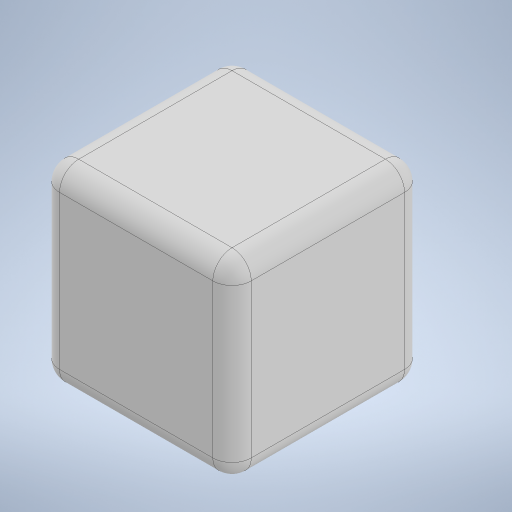
# Autodesk Inventor part: Holder
Saved by Autodesk Inventor 2023 (Build 270158000, 158)
## iProperties
Created: 2022-12-13
Part Number: Holder
Material: Generic
Document SubType Name: Modeling
Designer: romanp
Density: 1 g/cm^3
Appearance: Default
Author: romanp
Autodesk Inventor part; units mm, degrees
ref_plane "YZ Plane" through (0, 0, 0) normal (1, 0, 0) x (0, 1, 0)
ref_plane "XZ Plane" through (0, 0, 0) normal (0, 1, 0) x (-1, 0, 0)
ref_plane "XY Plane" through (0, 0, 0) normal (0, 0, 1) x (1, 0, 0)
sketch "Sketch5" plane through (0, 0, 0) normal (0, 0, 1) x (1, 0, 0)
  circle A0 centre (0, 0) radius 3.75
  dimension "d11" = 7.5
  constraints: 1 centre point, 1 coincident
  measures "d11" diameter of A0
extrude "Extrusion4" add sketch "Sketch5" along normal blind 5
sketch "Sketch6" plane through (0, 0, 5) normal (0, 0, 1) x (1, 0, 0)
  line L0 (0, 0) -> (-10, 0)
  line L1 (-10, 0) -> (-10, 10)
  line L2 (-10, 10) -> (10, 10)
  line L3 (10, 10) -> (10, -10)
  line L4 (10, -10) -> (-10, -10)
  line L5 (-10, -10) -> (-10, 0)
  dimension "d19" = 10
  dimension "d20" = 10
  dimension "d21" = 20
  dimension "d22" = 20
  dimension "d23" = 20
  constraints: 12 end point, 3 perpendicular, 1 collinear, 1 horizontal, 1 point on line
  measures "d19" distance of L0.start L0.end
  measures "d20" distance of L0.end L1.end
  measures "d21" distance of L1.end L2.end
  measures "d22" distance of L2.end L3.end
  measures "d23" distance of L3.end L4.end
extrude "Extrusion5" add sketch "Sketch6" along normal blind 20
fillet "Fillet1" radius 2 12 edges at (-10, 0, 5) (0, -10, 5) (-10, -10, 15) (0, 10, 5) (10, 10, 15) (10, 0, 5) (-10, 10, 15) (-10, 0, 25) (0, 10, 25) (10, 0, 25) (0, -10, 25) (10, -10, 15)
body "Solid2"
